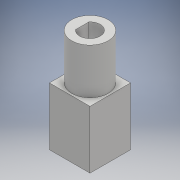
# Autodesk Inventor part: MotorConnectionmm
Saved by Autodesk Inventor 2017 (Build 210142000, 142)
## iProperties
Created: 2017-02-11
Part Number: MotorConnectionmm
Material: Generic
Document SubType Name: Modeling
Designer: aribu
Density: 1 g/cm^3
Appearance: Default
Author: aribu
Autodesk Inventor part; units mm, degrees
ref_plane "YZ Plane" through (0, 0, 0) normal (1, 0, 0) x (0, 1, 0)
ref_plane "XZ Plane" through (0, 0, 0) normal (0, 1, 0) x (-1, 0, 0)
ref_plane "XY Plane" through (0, 0, 0) normal (0, 0, 1) x (1, 0, 0)
sketch "Sketch1" plane through (0, 0, 0) normal (0, 0, 1) x (1, 0, 0)
  line L0 (-4.1693, 5.0958) -> (4.7207, 5.0958)
  line L1 (4.7207, 5.0958) -> (4.7207, -3.7942)
  line L2 (4.7207, -3.7942) -> (-4.1693, -3.7942)
  line L3 (-4.1693, -3.7942) -> (-4.1693, 5.0958)
  point P0 (0, 0)
  dimension "d0" = 8.89
  dimension "d1" = 8.89
  constraints: 8 end point, 2 parallel, 1 horizontal, 1 perpendicular
  measures "d0" distance of L0.start L0.end
  measures "d1" distance of L0.end L1.end
extrude "Extrusion1" add sketch "Sketch1" along normal blind 12.7
sketch "Sketch2" plane through (0, 0, 12.7) normal (0, 0, 1) x (1, 0, 0)
  circle A0 centre (0.2707, 0.6458) radius 4
  line L0 (-4.1693, 5.0958) -> (4.7207, 5.0958) projected
  line L1 (4.7207, -3.7942) -> (4.7207, 5.0958) projected
  arc A1 (-1.4293, -0.8282) -> (-1.4293, 2.1197) centre (0.2707, 0.6458) ccw
  line L2 (-1.4293, 2.1197) -> (-1.4293, -0.8282)
  point P0 (0, 0)
  dimension "d4" = 4.45
  dimension "d5" = 4.45
  dimension "d6" = 8
  dimension "d7" = 4.5
  dimension "d8" = 1.7
  constraints: 2 centre point, 2 end point, 2 point on circle, 1 coincident, 1 vertical
  measures "d4" distance from line of L0 A0.centre
  measures "d5" distance from line of L1 A0.centre
  measures "d6" diameter of A0
  measures "d7" diameter of A1
  measures "d8" distance from line of L2 A0.centre
extrude "Extrusion2" add sketch "Sketch2" along normal blind 10
body "Solid1"
